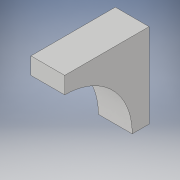
# Autodesk Inventor part: Ramp
Saved by Autodesk Inventor 2019 (Build 230136000, 136)
## iProperties
Created: 2020-01-13
Part Number: Ramp
Material: Generic
Document SubType Name: Modeling
Designer: james
Density: 1 g/cm^3
Appearance: Default
Author: james
Autodesk Inventor part; units mm, degrees
ref_plane "YZ Plane" through (0, 0, 0) normal (1, 0, 0) x (0, 1, 0)
ref_plane "XZ Plane" through (0, 0, 0) normal (0, 1, 0) x (-1, 0, 0)
ref_plane "XY Plane" through (0, 0, 0) normal (0, 0, 1) x (1, 0, 0)
sketch "Sketch1" plane through (0, 0, 0) normal (1, 0, 0) x (0, 1, 0)
  circle A0 centre (0, 1.3072) radius 101.6
  circle A1 centre (0, 1.3072) radius 107.95
  point P0 (0, 0)
  dimension "d0" = 203.2
  dimension "d1" = 215.9
  constraints: 2 centre point, 1 coincident
  measures "d0" diameter of A0
  measures "d1" diameter of A1
extrude "Extrusion1" add sketch "Sketch1" along normal blind 50.8
sketch "Sketch2" plane through (50.8, 0, 1.3072) normal (1, 0, 0) x (0, 0, -1)
  circle A0 centre (0, 0) radius 101.6 projected
  circle A1 centre (0, 0) radius 107.95 projected
  line L0 (127, 0) -> (127, 127)
  line L1 (127, 127) -> (0, 127)
  line L2 (0, 127) -> (0, 107.95)
  arc A2 (107.95, 0) -> (0, 107.95) centre (0, 0) ccw
  line L3 (107.95, 0) -> (127, 0)
  dimension "d13" = 127
  dimension "d15" = 127
  constraints: 8 end point, 4 point on circle, 2 parallel, 1 centre point, 1 coincident, 1 concentric, 1 horizontal, 1 perpendicular
  measures "d13" distance from line of A1.centre L1
  measures "d15" distance from line of A0.centre L0
extrude "Extrusion2" add sketch "Sketch2" against normal blind 50.8 contours A1 L2 L1 L0 L3
sketch "Sketch3" plane through (50.8, 0, 0) normal (1, 0, 0) x (0, 0, -1)
  line L0 (-164.0903, 142.5246) -> (-1.3072, 142.5246)
  line L1 (-20.2178, -157.5435) -> (-164.0903, -157.5435)
  line L2 (-164.0903, -157.5435) -> (-164.0903, 142.5246)
  line L3 (195.7449, 0) -> (-1.3072, 0)
  line L4 (-20.2178, -149.5335) -> (195.7449, -149.5335)
  line L5 (195.7449, -149.5335) -> (195.7449, 0)
  line L6 (106.6428, 0) -> (125.6928, 0) projected
  line L7 (-1.3072, 142.5246) -> (-1.3072, 0)
  line L8 (-20.2178, -149.5335) -> (-20.2178, -157.5435)
  line L9 (-1.3072, 127) -> (-1.3072, 107.95) projected
  point P0 (0, 0)
  dimension "d18" = 0
  dimension "d19" = 0
  constraints: 16 end point, 4 parallel, 2 horizontal, 2 perpendicular
  measures "d18" distance between parallel lines of L6 L3
  measures "d19" distance between parallel lines of L7 L9
extrude "Extrusion3" cut sketch "Sketch3" against normal blind 50.8
body "Solid1"
